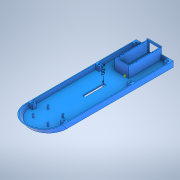
# Autodesk Inventor part: корпус
Saved by Autodesk Inventor 2022 (Build 260153000, 153)
## iProperties
Created: 2021-12-25
Part Number: корпус
Material: Пластик ПЭТ
Document SubType Name: Modeling
Designer: Grigori
Density: 1.541 g/cm^3
Appearance: Поликарбонат — прозрачный
Author: Grigori
Autodesk Inventor part; units mm, degrees
ref_plane "YZ Plane" through (0, 0, 0) normal (1, 0, 0) x (0, 1, 0)
ref_plane "XZ Plane" through (0, 0, 0) normal (0, 1, 0) x (-1, 0, 0)
ref_plane "XY Plane" through (0, 0, 0) normal (0, 0, 1) x (1, 0, 0)
sketch "Эскиз1" plane through (0, 0, 0) normal (0, 1, 0) x (-1, 0, 0)
  line L0 (250, 0) -> (50, 0)
  arc A0 (250, 400) -> (50, 400) centre (150, 400) ccw
  line L1 (50, 400) -> (50, 0)
  line L2 (250, 400) -> (250, 0)
  point P0 (0, 0)
  point P1 (150, 600)
  constraints: 6 end point, 2 perpendicular, 2 point on circle, 1 centre point, 1 tangent
ref_plane "РабПлоскость2" through (0, -30, 400) normal (0, 1, 0) x (0, 0, -1)
sketch "Эскиз5" plane through (0, -30, 400) normal (0, 1, 0) x (0, 0, -1)
  arc A0 (25, 250) -> (25, 50) centre (25, 150) ccw
  line L0 (25, 250) -> (400, 250)
  line L1 (25, 50) -> (400, 50)
  line L2 (400, 50) -> (400, 250)
  point P0 (400, 0)
  point P1 (0, 0)
  point P2 (150, 600)
  constraints: 6 end point, 2 horizontal, 2 point on circle, 1 centre point, 1 vertical
loft "Лофт2" add profiles "Эскиз1", "Эскиз5"
shell "Оболочка2" thickness 5 removed faces 1 at (-116.6667, 0, 266.6667)
sketch "Эскиз6" plane through (-245, -25, 5) normal (0, 1, 0) x (1, 0, 0)
  line L0 (190, 0) -> (190, -395) projected
  line L1 (190, 0) -> (170, 0)
  line L2 (170, 0) -> (170, -20)
  line L3 (170, -20) -> (190, -20)
  line L4 (190, -20) -> (190, 0)
  line L5 (0, 0) -> (190, 0) projected
  line L6 (0, 0) -> (20, 0)
  line L7 (20, 0) -> (20, -20)
  line L8 (20, -20) -> (0, -20)
  line L9 (0, -20) -> (0, 0)
  line L10 (0, -395) -> (0, 0) projected
  line L11 (20, -20) -> (380, -20) construction
  line L12 (170, -20) -> (530, -20) construction
  line L13 (170, -380) -> (190, -380)
  line L14 (190, -380) -> (190, -360)
  line L15 (190, -360) -> (170, -360)
  line L16 (170, -360) -> (170, -380)
  line L17 (20, -380) -> (0, -380)
  line L18 (0, -380) -> (0, -360)
  line L19 (0, -360) -> (20, -360)
  line L20 (20, -360) -> (20, -380)
  point P0 (245, 5)
  dimension "d31" = 20
  dimension "d32" = 20
  dimension "d33" = 20
  dimension "d34" = 20
  dimension "d36" = 360
  dimension "d38" = 360
  dimension "d40" = 20
  dimension "d41" = 20
  dimension "d42" = 20
  dimension "d43" = 20
  constraints: 36 end point, 8 parallel, 6 horizontal, 4 perpendicular
  measures "d31" distance of L3.end L2.end
  measures "d32" distance of L2.end L1.end
  measures "d33" distance of L7.end L8.end
  measures "d34" distance of L6.end L7.end
  measures "d36" distance of L7.end L17.start
  measures "d38" distance of L2.end L13.start
  measures "d40" distance of L15.end L14.end
  measures "d41" distance of L14.end L13.end
  measures "d42" distance of L18.end L19.end
  measures "d43" distance of L17.end L18.end
extrude "Выдавливание3" add sketch "Эскиз6" along normal blind 25
sketch "Эскиз7" plane through (-150, 0, 400) normal (0, 1, 0) x (1, 0, 0)
  line L0 (75, 375) -> (95, 375) projected
  line L1 (75, 395) -> (75, 375) projected
  line L2 (-75, 375) -> (-75, 395) projected
  line L3 (-95, 375) -> (-75, 375) projected
  line L4 (-75, 35) -> (-95, 35) projected
  line L5 (-75, 15) -> (-75, 35) projected
  line L6 (75, 35) -> (75, 15) projected
  line L7 (95, 35) -> (75, 35) projected
  circle A0 centre (85, 25) radius 5
  circle A1 centre (-85, 25) radius 5
  circle A2 centre (-85, 385) radius 5
  circle A3 centre (85, 385) radius 5
  point P0 (150, 400)
  dimension "d46" = 10
  dimension "d47" = 10
  dimension "d48" = 10
  dimension "d49" = 10
  constraints: 4 centre point
  measures "d46" diameter of A0
  measures "d47" diameter of A1
  measures "d48" diameter of A2
  measures "d49" diameter of A3
extrude "Выдавливание4" cut sketch "Эскиз7" against normal through all
thread "Резьба1" size "M10x1.5" class "6H" standard "ANSI Metric M Profile" full length
thread "Резьба2" size "M10x1.5" class "6H" standard "ANSI Metric M Profile" full length
thread "Резьба3" size "M10x1.5" class "6H" standard "ANSI Metric M Profile" full length
thread "Резьба4" size "M10x1.5" class "6H" standard "ANSI Metric M Profile" full length
sketch "Эскиз11" plane through (-150, 0, 400) normal (0, 1, 0) x (1, 0, 0)
  line L0 (-75, 395) -> (75, 395) projected
  line L1 (75, 395) -> (-75, 395)
  line L2 (-75, 395) -> (-75, 400)
  line L3 (-75, 400) -> (75, 400)
  line L4 (75, 400) -> (75, 395)
  point P0 (150, 400)
  dimension "d62" = 150
  dimension "d63" = 5
  constraints: 8 end point, 2 parallel, 1 horizontal, 1 perpendicular
  measures "d62" distance of L2.end L3.end
  measures "d63" distance of L1.end L2.end
extrude "Выдавливание5" cut sketch "Эскиз11" against normal blind 25
move faces "Перенос1" translate (0, 0, -200) faces at (-125, -28.3333, 0)
sketch "Эскиз13" plane through (-150, 0, 400) normal (0, 1, 0) x (1, 0, 0)
  line L0 (95, 395) -> (95, 600)
  line L1 (100, 600) -> (-100, 600) projected
  line L2 (75, 395) -> (95, 395)
  line L3 (75, 395) -> (75, 600)
  line L4 (75, 600) -> (95, 600)
  line L5 (-95, 395) -> (-95, 600)
  line L6 (-75, 395) -> (-95, 395)
  line L7 (-75, 395) -> (-75, 600)
  line L8 (-75, 600) -> (-95, 600)
  point P0 (150, 400)
  point P1 (95, 375)
  point P2 (75, 375)
  constraints: 16 end point, 2 perpendicular, 1 point on line, 1 vertical
extrude "Выдавливание6" cut sketch "Эскиз13" against normal blind 25
sketch "Эскиз14" plane through (-245, -25, 25) normal (0, 1, 0) x (1, 0, 0)
  line L0 (195, 225) -> (-5, 225) projected
  line L1 (195, 225) -> (-5, 225)
  line L2 (-5, 225) -> (-5, 220)
  line L3 (-5, 225) -> (-5, -350) projected
  line L4 (-5, 220) -> (195, 220)
  line L5 (195, -350) -> (195, 225) projected
  point P0 (245, 25)
  dimension "d76" = 5
  constraints: 6 end point, 2 point on line, 1 collinear, 1 perpendicular
  measures "d76" distance of L0.end L2.end
extrude "Выдавливание7" add sketch "Эскиз14" along normal blind 25
sketch "Эскиз15" plane through (-150, 0, 400) normal (0, 1, 0) x (1, 0, 0)
  line L0 (-95, 395) -> (-95, 595) projected
  line L1 (-95, 595) -> (-75, 595)
  line L2 (-75, 595) -> (-75, 575)
  line L3 (-75, 575) -> (-95, 575)
  line L4 (-95, 575) -> (-95, 595)
  line L5 (95, 595) -> (95, 395) projected
  line L6 (95, 595) -> (75, 595)
  line L7 (75, 595) -> (75, 575)
  line L8 (75, 575) -> (95, 575)
  line L9 (95, 575) -> (95, 595)
  point P0 (150, 400)
  dimension "d79" = 20
  dimension "d80" = 20
  dimension "d81" = 20
  dimension "d82" = 20
  constraints: 16 end point, 4 parallel, 2 horizontal, 2 perpendicular
  measures "d79" distance of L2.end L3.end
  measures "d80" distance of L1.end L2.end
  measures "d81" distance of L8.end L7.end
  measures "d82" distance of L7.end L6.end
extrude "Выдавливание8" add sketch "Эскиз15" against normal through all
sketch "Эскиз16" plane through (-150, 0, 400) normal (0, 1, 0) x (1, 0, 0)
  line L0 (-95, 575) -> (-75, 575) projected
  line L1 (-75, 575) -> (-75, 595) projected
  line L2 (75, 595) -> (75, 575) projected
  line L3 (75, 575) -> (95, 575) projected
  circle A0 centre (-85, 585) radius 5
  circle A1 centre (85, 585) radius 5
  point P0 (150, 400)
  dimension "d85" = 10
  dimension "d86" = 10
  constraints: 2 centre point
  measures "d85" diameter of A0
  measures "d86" diameter of A1
extrude "Выдавливание9" cut sketch "Эскиз16" against normal through all
thread "Резьба5" size "M10x1.5" class "6H" standard "ANSI Metric M Profile" full length
thread "Резьба6" size "M10x1.5" class "6H" standard "ANSI Metric M Profile" full length
sketch "Эскиз17" plane through (-245, -25, 25) normal (0, 1, 0) x (1, 0, 0)
  line L0 (95, 225) -> (127.5, 225)
  line L1 (95, 225) -> (62.5, 225)
  line L2 (62.5, 225) -> (62.5, 220)
  line L3 (62.5, 225) -> (67.5, 225) construction
  line L4 (62.5, 220) -> (127.5, 220)
  line L5 (127.5, 225) -> (127.5, 220)
  point P0 (245, 25)
  point P1 (62.5, 222.5)
  point P2 (127.5, 222.5)
  dimension "d94" = 32.5
  dimension "d103" = 32.5
  dimension "d104" = 5
  dimension "d105" = 90
  constraints: 12 end point, 2 perpendicular, 1 horizontal, 1 vertical
  measures "d94" distance of L0.start L0.end
  measures "d103" distance of L0.start L1.end
  measures "d104" distance of L1.end L2.end
  measures "d105" angle of L2 L3
extrude "Выдавливание11" cut sketch "Эскиз17" along normal through all
sketch "Эскиз19" plane through (-50, -30, -200) normal (0, 0, -1) x (-1, 0, 0)
  line L0 (67.5, 5) -> (67.5, 30) projected
  line L1 (67.5, 5) -> (67.5, 62)
  line L2 (67.5, 5) -> (124.5, 5) construction
  line L3 (132.5, 5) -> (67.5, 5) projected
  line L4 (132.5, 5) -> (132.5, 62)
  line L5 (132.5, 30) -> (132.5, 5) projected
  line L6 (132.5, 5) -> (189.5, 5) construction
  line L7 (132.5, 62) -> (67.5, 62)
  line L8 (67.5, 67) -> (62.5, 67)
  line L9 (62.5, 67) -> (62.5, 5)
  line L10 (25, 5) -> (67.5, 5) projected
  line L11 (132.5, 5) -> (137.5, 5)
  line L12 (132.5, 5) -> (175, 5) projected
  line L13 (67.5, 67) -> (137.5, 67)
  line L14 (137.5, 67) -> (137.5, 5)
  point P0 (-50, 30)
  dimension "d108" = 57
  dimension "d109" = 90
  dimension "d110" = 57
  dimension "d111" = 90
  dimension "d112" = 5
  dimension "d113" = 5
  dimension "d114" = 5
  constraints: 20 end point, 4 perpendicular, 3 horizontal, 2 collinear, 2 point on line
  measures "d108" distance of L0.start L1.end
  measures "d109" angle of L2 L1
  measures "d110" distance of L3.start L4.end
  measures "d111" angle of L6 L4
  measures "d112" distance of L1.end L8.start
  measures "d113" distance of L8.start L8.end
  measures "d114" distance of L3.start L11.end
extrude "Выдавливание12" add sketch "Эскиз19" against normal blind 5 contours L10 L9 L8 L13 L14 L11 L4 L7 L1 L0
sketch "Эскиз20" plane through (-50, -30, -200) normal (0, 0, -1) x (-1, 0, 0)
  line L0 (67.5, 5) -> (67.5, 62) projected
  line L1 (67.5, 62) -> (132.5, 62) projected
  line L2 (128.5, 58) -> (71.5, 58)
  line L3 (71.5, 58) -> (71.5, 9)
  line L4 (71.5, 9) -> (128.5, 9)
  line L5 (128.5, 9) -> (128.5, 58)
  line L6 (132.5, 5) -> (67.5, 5) projected
  line L7 (132.5, 62) -> (132.5, 5) projected
  point P0 (-50, 30)
  constraints: 8 end point, 2 parallel, 1 horizontal, 1 perpendicular
extrude "Выдавливание13" add sketch "Эскиз20" against normal blind 5
sketch "Эскиз21" plane through (-245, -25, 25) normal (0, 1, 0) x (1, 0, 0)
  line L0 (132.5, 220) -> (57.5, 220) projected
  line L1 (95, 52) -> (127.5, 52)
  line L2 (95, 52) -> (62.5, 52)
  line L3 (62.5, 52) -> (62.5, 220)
  line L4 (127.5, 52) -> (127.5, 220)
  line L5 (62.5, 47) -> (57.5, 47)
  line L6 (132.5, 220) -> (170, 220) projected
  line L7 (57.5, 47) -> (132.5, 47)
  line L8 (132.5, 47) -> (132.5, 220)
  line L9 (132.5, 220) -> (57.5, 220)
  line L10 (57.5, 220) -> (57.5, 47)
  line L11 (127.5, 220) -> (132.5, 220)
  line L12 (57.5, 220) -> (62.5, 220)
  point P0 (245, 25)
  point P1 (62.5, 47)
  dimension "d124" = 32.5
  dimension "d126" = 5
  dimension "d127" = 5
  constraints: 22 end point, 3 perpendicular, 2 collinear, 2 horizontal, 2 parallel, 2 point on line
  measures "d124" distance of L1.start L1.end
  measures "d126" distance of L2.end L5.start
  measures "d127" distance of L5.start L5.end
extrude "Выдавливание14" add sketch "Эскиз21" along normal blind 57 contours L8 L7 L5 L10 L0 L3 L2 L1 L4
sketch "Эскиз22" plane through (-112.5, 0, -200) normal (1, 0, 0) x (0, 0, -1)
  point P0 (-200, 0)
sketch "Эскиз24" plane through (-245, 32, 25) normal (0, 1, 0) x (1, 0, 0)
  circle A0 centre (130, 197.5) radius 1.5
  circle A1 centre (130, 177.5) radius 1.5
  circle A2 centre (130, 69.5) radius 1.5
  circle A3 centre (130, 89.5) radius 1.5
  circle A4 centre (60, 197.5) radius 1.5
  circle A5 centre (60, 177.5) radius 1.5
  circle A6 centre (60, 89.5) radius 1.5
  circle A7 centre (60, 69.5) radius 1.5
  point P0 (245, 25)
  dimension "d130" = 3
  dimension "d131" = 3
  constraints: 8 centre point
  measures "d130" diameter of A0
  measures "d131" diameter of A1
extrude "Выдавливание15" cut sketch "Эскиз24" against normal blind 5
thread "Резьба7" size "M3x0.5" class "6H" standard "ANSI Metric M Profile" full length
thread "Резьба8" size "M3x0.5" class "6H" standard "ANSI Metric M Profile" full length
thread "Резьба9" size "M3x0.5" class "6H" standard "ANSI Metric M Profile" full length
thread "Резьба10" size "M3x0.5" class "6H" standard "ANSI Metric M Profile" full length
thread "Резьба11" size "M3x0.5" class "6H" standard "ANSI Metric M Profile" full length
thread "Резьба12" size "M3x0.5" class "6H" standard "ANSI Metric M Profile" full length
thread "Резьба13" size "M3x0.5" class "6H" standard "ANSI Metric M Profile" full length
thread "Резьба14" size "M3x0.5" class "6H" standard "ANSI Metric M Profile" full length
sketch "Эскиз27" plane through (-245, -25, 365) normal (0, 1, 0) x (1, 0, 0)
  circle A0 centre (55, 28) radius 5
  line L0 (20, -20) -> (20, 0) projected
  line L1 (20, 0) -> (0, 0) projected
  circle A1 centre (135, 28) radius 5
  line L2 (170, 0) -> (170, -20) projected
  line L3 (190, 0) -> (170, 0) projected
  circle A2 centre (55, -52) radius 5
  circle A3 centre (135, -52) radius 5
  point P0 (245, 365)
  dimension "d150" = 10
  dimension "d151" = 35
  dimension "d152" = 28
  dimension "d153" = 10
  dimension "d154" = 35
  dimension "d155" = 28
  dimension "d156" = 10
  dimension "d157" = 10
  dimension "d158" = 90
  dimension "d159" = 90
  dimension "d161" = 35
  dimension "d164" = 80
  constraints: 4 centre point
  measures "d150" diameter of A0
  measures "d151" distance from line of A0.centre L0
  measures "d152" distance from line of L1 A0.centre
  measures "d153" diameter of A1
  measures "d154" distance from line of L2 A1.centre
  measures "d155" distance from line of L3 A1.centre
  measures "d156" diameter of A2
  measures "d157" diameter of A3
  measures "d161" distance from line of L0 A2.centre
  measures "d164" distance of A3.centre A2.centre
extrude "Выдавливание16" add sketch "Эскиз27" along normal blind 15
sketch "Эскиз28" plane through (-245, -25, 365) normal (0, 1, 0) x (1, 0, 0)
  line L0 (190, 340) -> (190, 0) projected
  line L1 (0, 0) -> (0, 340) projected
  line L2 (101.8, 295.6) -> (88.2, 295.6)
  line L3 (88.2, 295.6) -> (88.2, 182)
  line L4 (88.2, 182) -> (101.8, 182)
  line L5 (101.8, 182) -> (101.8, 295.6)
  line L6 (101.8, 295.6) -> (88.2, 182) construction
  line L7 (88.2, 295.6) -> (101.8, 182) construction
  point P0 (245, 365)
  point P1 (95, 238.8)
  dimension "d167" = 190
  dimension "d168" = 113.6
  dimension "d169" = 13.6
  dimension "d170" = 95
  constraints: 12 end point, 2 midpoint, 2 parallel, 1 horizontal, 1 perpendicular
  measures "d167" distance between parallel lines of L0 L1
  measures "d168" distance of L2.end L3.end
  measures "d169" distance of L2.start L2.end
  measures "d170" distance from line of point (95, 238.8) L1
extrude "Выдавливание17" cut sketch "Эскиз28" against normal through all
